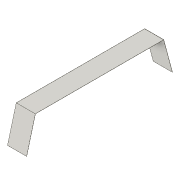
# Autodesk Inventor part: Fender
Saved by Autodesk Inventor 2018 (Build 220112000, 112)
## iProperties
Created: 2017-07-14
Part Number: Fender
Material: Generic
Document SubType Name: Modeling
Designer: thoma
Density: 1 g/cm^3
Appearance: Steel
Author: thoma
Autodesk Inventor part; units mm, degrees
ref_plane "YZ Plane" through (0, 0, 0) normal (1, 0, 0) x (0, 1, 0)
sketch "Sketch1" plane through (0, 0, 0) normal (1, 0, 0) x (0, 1, 0)
  line L0 (-433.6974, 970.2859) -> (-433.6974, 972.2502)
  line L1 (-433.6974, 972.2502) -> (0, 856.0414)
  line L2 (0, 856.0414) -> (0, -856.0414)
  line L3 (0, -856.0414) -> (-433.6974, -972.2502)
  line L4 (-433.6974, -972.2502) -> (-433.6974, -970.2859)
  line L5 (-433.6974, -970.2859) -> (-1.8974, -854.5855)
  line L6 (-1.8974, -854.5855) -> (-1.8974, 854.5855)
  line L7 (-1.8974, 854.5855) -> (-433.6974, 970.2859)
  point P0 (0, 0)
  point P1 (-217.7974, 914.4)
  point P2 (-217.7974, -914.4)
  point P3 (0, 0)
  dimension "d6" = 433.6974
  dimension "d7" = 1.8974
  dimension "d8" = 1.8974
  dimension "d9" = 105
  dimension "d10" = 217.7974
  dimension "d11" = 217.7974
  dimension "d12" = 1828.8
  dimension "d15" = 1940.5718
  constraints: 16 end point, 4 parallel, 4 point on line, 2 equal length, 1 coincident, 1 midpoint, 1 vertical
  measures "d6" distance between parallel lines of L0 L2
  measures "d7" distance between parallel lines of L1 L7
  measures "d8" distance between parallel lines of L2 L6
  measures "d9" angle of L7 L6
  measures "d10" distance from line of L2 point (-217.797, 914.4)
  measures "d11" distance from line of L2 point (-217.797, -914.4)
  measures "d12" distance of point (-217.797, 914.4) point (-217.797, -914.4)
  measures "d15" distance of L4.end L0.start
extrude "Extrusion1" add sketch "Sketch1" against normal blind 254
ref_plane "Work Plane1" through (0, -433.6974, 970.2859) normal (0, -1, 0) x (-1, 0, 0)
ref_plane "Work Plane2" through (0, -433.6974, -970.2859) normal (0, 0, 1) x (1, 0, 0)
body "Solid1"
